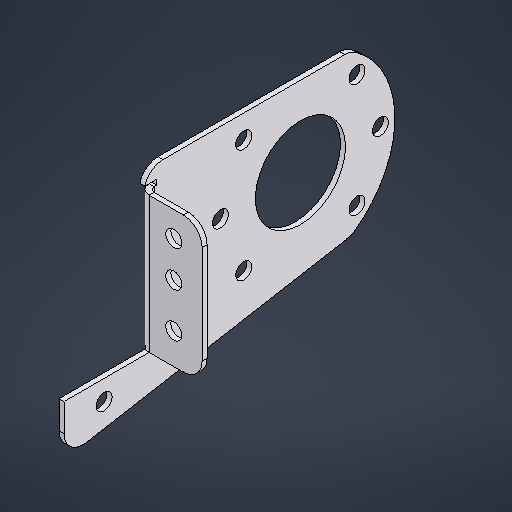
# Autodesk Inventor part: INSIDE_INTAKE_PLATE_MOTOR_MOUNT
Saved by Autodesk Inventor 2026.1 (Build 301233020, 233B)
## iProperties
Created: 2026-04-02
Part Number: INSIDE_INTAKE_PLATE_MOTOR_MOUNT
Material: Aluminum, 6061-T6
Document SubType Name: Sheet Metal
Designer: 4aida
Density: 2.71 g/cm^3
Sheet Metal Rule: Default_mm
Appearance: Metal-AL-6061 (Flat)
Mass: 46.2037 g
Surface Area: 122.322 cm^2
Volume: 17.0493 cm^3
Flat Pattern Width: 6.04625 cm
Flat Pattern Length: 10.9906 cm
Flat Pattern Area: 66.4519 cm^2
Sheet Metal Width: 60.463 mm
Sheet Metal Length: 109.906 mm
Sheet Metal Area: 6645.189 mm^2
Author: 4aida
Autodesk Inventor part; units mm, degrees
note: some values were not read from the file. Chosen so that the rebuilt part matches the saved one: relief shape of "Plate2".
ref_plane "YZ Plane" through (0, 0, 0) normal (1, 0, 0) x (0, 1, 0)
ref_plane "XZ Plane" through (0, 0, 0) normal (0, 1, 0) x (-1, 0, 0)
ref_plane "XY Plane" through (0, 0, 0) normal (0, 0, 1) x (1, 0, 0)
sketch "Sketch1" plane through (0, 0, 0) normal (1, 0, 0) x (0, 1, 0)
  line L0 (-39.3892, -105) -> (-110, -20.8494)
  line L1 (-110, -20.8494) -> (-110, 0)
  line L2 (-110, 0) -> (0, 0)
  line L3 (0, 0) -> (0, -105)
  line L4 (0, -105) -> (-39.3892, -105)
  line L5 (-110, -20.8494) -> (-119.38, 0) construction
  line L6 (-119.38, 0) -> (-110, 0) construction
  line L7 (-50.8, -25.4) -> (0, -25.4) construction
  line L8 (0, -25.4) -> (0, 0) construction
  line L9 (0, 0) -> (-50.8, 0) construction
  line L10 (-50.8, 0) -> (-50.8, -25.4) construction
  line L11 (-50.8, -25.4) -> (0, 0) construction
  line L12 (0, -25.4) -> (-50.8, 0) construction
  circle A0 centre (-12.7, -12.7) radius 3
  circle A1 centre (-38.1, -12.7) radius 3
  circle A2 centre (-25.4, -75) radius 14.2875
  circle A3 centre (-25.4, -75) radius 30
  line L13 (-50.8, -90.9637) -> (-50.8, -59.0363)
  line L14 (-50.8, -25.4) -> (0, -25.4)
  line L15 (-66.8394, 0) -> (-50.8, -90.9637)
  line L16 (-50.8, -25.4) -> (-50.8, 0)
  point P0 (-25.4, -12.7)
  point P1 (-25.4, -25.4)
  point P2 (-50.8, -75)
  point P3 (0, -90.9637)
  point P4 (0, -25.4)
  point P5 (-50.8, 0)
  dimension "d0" = 50
  dimension "d1" = 119.38
  dimension "d2" = 50.8
  dimension "d3" = 25.4
  dimension "d4" = 25.4
  dimension "d5" = 12.7
  dimension "d6" = 6
  dimension "d7" = 6
  dimension "d11" = 75
  dimension "d13" = 110
  dimension "d16" = 60
  dimension "d17" = 25.4
  dimension "d18" = 25.4
  dimension "d31" = 28.575
  dimension "d33" = 10
  measures "d0" angle of L0 L2
  measures "d1" distance from line of L3 L5.end
  measures "d2" distance of L7.start L7.end
  measures "d3" distance of L9.end L7.start
  measures "d4" distance of A1.centre A0.centre
  measures "d5" distance of point (-25.4, -12.7) A0.centre
  measures "d6" diameter of A0
  measures "d7" diameter of A1
  measures "d11" distance from line of A2.centre L9
  measures "d13" distance between parallel lines of L3 L1
  measures "d16" diameter of A3
  measures "d17" distance from line of A2.centre L3
  measures "d18" distance of point (-50.8, -75) A2.centre
  measures "d31" diameter of A2
  measures "d33" angle of L13 L15
extrude "Plate1" add sketch "Sketch1" along normal blind 1.5875 contours A3 L13 L3 | L15 A3 L13 | L15 L2 L16 L14 L3 A3
fillet "Corner Round2" radius 6 4 edges at (0.7937, 0, -90.9637) (0.7937, -50.8, -90.9637) (0.7937, 0, -25.4) (0.7937, -66.8394, 0)
sketch "Sketch3" plane through (0, -50.8, -26.9875) normal (0, 0, 1) x (1, 0, 0)
  line L0 (0, 44.8) -> (0, 1.5875)
  line L1 (0, 1.5875) -> (20, 1.5875)
  line L2 (20, 1.5875) -> (20, 44.8)
  line L3 (20, 44.8) -> (0, 44.8)
  constraints: 8 end point
edge flange "Flange1" height 20 angle 90 thickness 1.5875 bend radius 1.5875 thickness toward (0, 0, 1) relief straight relief width 1.5875 relief depth 0.7937 edges at (1.5875, -28.4, -25.4) wall of the first edge with corners at (0, -6, -26.9875) (0, -49.2125, -26.9875) (20, -49.2125, -26.9875) (20, -6, -26.9875)
bend "Bend1"
corner "Corner1"
sketch "Sketch4" plane through (1.5875, 0, 0) normal (1, 0, 0) x (0, 0, -1)
  circle A0 centre (75, -25.4) radius 14.2875 projected
  point P0 (0, 0)
  point P1 (100.4, -25.4)
  point P2 (92.9605, -7.4395)
  point P3 (75, 0)
  point P4 (57.0395, -7.4395)
  point P5 (49.6, -25.4)
  point P6 (57.0395, -43.3605)
  point P7 (75, -50.8)
  point P8 (92.9605, -43.3605)
  dimension "d45" = 25.4
  dimension "d48" = 360
  constraints: 1 horizontal alignment, 9 other
  measures "d45" distance of A0.centre point (100.4, -25.4)
hole "Hole2" at (1.5875, -25.4, -100.4) at (1.5875, -7.4395, -92.9605) at (1.5875, -7.4395, -57.0395) at (1.5875, -25.4, -49.6) at (1.5875, -43.3605, -57.0395) at (1.5875, -43.3605, -92.9605) direction (-1, 0, 0) diameter 5.105 depth 1.5875 tip angle 118 clearance for "Flat Head Machine Screw (82)" size "#10" standard "Ansi Unified Screw Threads"
sketch "Sketch5" plane through (20, -49.2125, -26.9875) normal (0, 0, -1) x (-1, 0, 0)
  line L0 (0, 0) -> (16.825, 0) projected
  line L1 (16.825, 0) -> (16.825, 43.2125) projected
  point P0 (20, 49.2125)
  point P1 (8.9807, 9.8425)
  point P2 (8.9807, 35.2425)
  point P3 (8.4125, 0)
  point P4 (8.9807, 23.8125)
  dimension "d57" = 25.4
  dimension "d58" = 9.8425
  dimension "d67" = 23.8125
  dimension "d68" = 7.8443
  constraints: 2 vertical alignment, 1 midpoint
  measures "d57" distance of point (8.981, 35.242) point (8.981, 9.842)
  measures "d58" distance from line of L0 point (8.981, 9.842)
  measures "d67" distance from line of L0 point (8.981, 23.812)
  measures "d68" distance from line of L1 point (8.981, 9.842)
hole "Hole3" at (11.0193, -39.37, -26.9875) at (11.0193, -13.97, -26.9875) at (11.0193, -25.4, -26.9875) direction (0, 0, 1) diameter 5.105 end through all clearance for "Flat Head Machine Screw (82)" size "#10" standard "Ansi Unified Screw Threads"
fillet "Corner Round3" radius 6 2 edges at (20, -49.2125, -26.1938) (20, -6, -26.1937)
sketch "Sketch6" plane through (1.5875, 0, 0) normal (1, 0, 0) x (0, 0, -1)
  line L0 (29.3688, -50.8) -> (0, -50.8) projected
  line L1 (0, -59.6888) -> (0, -50.8) projected
  point P0 (0, 0)
  point P1 (12.7, -57.15)
  dimension "d69" = 6.35
  dimension "d70" = 12.7
  measures "d69" distance from line of L0 point (12.7, -57.15)
  measures "d70" distance from line of point (12.7, -57.15) L1
hole "Hole4" at (1.5875, -57.15, -12.7) direction (-1, 0, 0) diameter 5.105 end through all clearance for "Flat Head Machine Screw (82)" size "#10" standard "Ansi Unified Screw Threads"
equation "\"d5\" = 0.5 * d4"
equation "\"d7\" = d6"
equation "\"d55\" = Thickness"
equation "\"d76\" = Thickness"
equation "\"d14\" = Thickness"
equation "\"d35\" = BendReliefWidth"
equation "\"d36\" = BendReliefDepth"
equation "\"d37\" = MinimumRemnant"
equation "\"d38\" = TransitionRadius"
equation "\"d41\" = BendRadius"
equation "\"d42\" = CornerReliefSize"
equation "\"d43\" = GapSize"
equation "\"d44\" = JacobiRadiusSize"
equation "\"d18\" = d17"
equation "\"BendRadius\" = Thickness"
equation "\"BendReliefWidth\" = Thickness"
equation "\"BendReliefDepth\" = 0.5 * Thickness"
equation "\"CornerReliefSize\" = 4 * Thickness"
equation "\"MinimumRemnant\" = 2 * Thickness"
equation "\"TransitionRadius\" = BendRadius"
equation "\"JacobiRadiusSize\" = BendRadius"
equation "\"GapSize\" = Thickness"
equation "\"Thickness\" = 1.5875"
body "Solid1"
